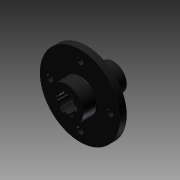
# Autodesk Inventor part: Denso-6
Saved by Autodesk Inventor 2011 (Build 150239000, 239)
## iProperties
Shininess: 64.0
Length Units: 11272
Angle Units: 11279
Time Units: 11290
Mass Units: 11286
Length Display Precision: 3
Angle Display Precision: 2
Category: Motors
Created: 2007-12-05
Material: ABS Plastic
Document SubType Name: Modeling
Density: 1 g/cm^3
Project: FIRST
Description: Coupler for Denso 6 Tooth Motor
Vendor: Pelham Plastics
Part Number: Denso-6
Density: 0.0
Volumn: 0.0
Area: 0.0
PropertySet Name: Model Information
Control State: 0
Master: False
Checked Out: False
Title: Coupler, Denso 6 tooth
Author: Autodesk, Inc.
Autodesk Inventor part; units mm, degrees
ref_plane "YZ Plane" through (0, 0, 0) normal (1, 0, 0) x (0, 1, 0)
ref_plane "XZ Plane" through (0, 0, 0) normal (0, 1, 0) x (-1, 0, 0)
ref_plane "XY Plane" through (0, 0, 0) normal (0, 0, 1) x (1, 0, 0)
sketch "Sketch1" plane through (0, 0, 0) normal (0, 0, 1) x (1, 0, 0)
  circle A0 centre (0, 0) radius 38.1
  dimension "d2" = 76.2
  constraints: 1 centre point
  measures "d2" diameter of A0
extrude "Extrusion1" add sketch "Sketch1" along normal mid plane 6.35
sketch "Sketch2" plane through (0, 0, 3.175) normal (0, 0, 1) x (1, 0, 0)
  circle A0 centre (0, 0) radius 38.1 projected
  point P0 (0, 28.575)
  dimension "d3" = 0
  dimension "d4" = 28.575
  measures "d3" horizontal distance of A0.centre point (0, 28.575)
  measures "d4" distance of A0.centre point (0, 28.575)
hole "Mounting Hole" at (0, 28.575, 3.175) direction (0, 0, -1) diameter 6.35 end through all
pattern_circular "Circular Pattern1" count 4 over 360 about axis through (0, 0, 0) along (0, 0, 1) of "Mounting Hole"
sketch "Sketch3" plane through (0, 0, 3.175) normal (0, 0, 1) x (1, 0, 0)
  circle A0 centre (0, 0) radius 38.1 projected
  circle A1 centre (0, 0) radius 15.875
  dimension "d15" = 31.75
  constraints: 1 centre point, 1 coincident
  measures "d15" diameter of A1
extrude "Extrusion2" add sketch "Sketch3" along normal blind 12.7 contours A1
sketch "Sketch8" plane through (0, 0, 15.875) normal (0, 0, 1) x (1, 0, 0)
  circle A0 centre (0, 0) radius 15.875 projected
  constraints: 1 coincident
hole "Hole3" at (0, 0, 15.875) direction (0, 0, -1) diameter 16.2 depth 14.986
sketch "Sketch4" plane through (0, 0, 15.875) normal (0, 0, 1) x (1, 0, 0)
  arc A0 (-3.0359, 9.528) -> (-6.5275, 7.5757) centre (0, 0) ccw
  circle A1 centre (0, 0) radius 15.875 projected
  line L0 (0, 0) -> (-5, 8.6603) construction
  line L1 (0, 0) -> (-10.16, 0) construction
  line L2 (-2.058, 7.8342) -> (-3.0359, 9.528)
  line L3 (-5.5564, 5.8937) -> (-6.5275, 7.5757)
  arc A2 (-2.058, 7.8342) -> (-5.5564, 5.8937) centre (0, 0) ccw
  circle A3 centre (0, 0) radius 8.1 projected
  dimension "d46" = 60
  dimension "d47" = 4
  dimension "d48" = 20
  constraints: 9 end point, 7 point on circle, 2 centre point, 2 parallel, 1 coincident, 1 concentric, 1 horizontal
  measures "d46" angle of L1 L0
  measures "d47" distance between parallel lines of L2 L3
  measures "d48" diameter of A0
extrude "Extrusion3" cut sketch "Sketch4" against normal up to surface (14.986 mm away) contours L2 A2 L3 A0
pattern_circular "Circular Pattern2" count 6 over 360 about axis through (0, 0, 0) along (0, 0, 1) of "Extrusion3"
sketch "Sketch5" plane through (0, 0, -3.175) normal (0, 0, -1) x (-1, 0, 0)
  circle A0 centre (0, 0) radius 38.1 projected
  circle A1 centre (0, 0) radius 14.9225
  dimension "d27" = 29.845
  constraints: 1 centre point, 1 coincident
  measures "d27" diameter of A1
extrude "Extrusion4" add sketch "Sketch5" along normal blind 25.4 draft -5 contours A1
sketch "Sketch6" plane through (0, 0, -28.575) normal (0, 0, -1) x (-1, 0, 0)
  circle A0 centre (0, 0) radius 12.7003 projected
  arc A1 (2.3812, -7.6374) -> (-2.3813, -7.6374) centre (0, 0) ccw
  line L0 (-2.3813, -7.6374) -> (-2.3812, -10.3188)
  line L1 (-2.3812, -10.3188) -> (2.3813, -10.3188)
  line L2 (2.3813, -10.3188) -> (2.3812, -7.6374)
  dimension "d31" = 16
  dimension "d32" = 4.7625
  dimension "d33" = 10.3187
  constraints: 6 end point, 2 parallel, 2 point on circle, 1 centre point, 1 coincident, 1 perpendicular, 1 vertical
  measures "d31" diameter of A1
  measures "d32" distance of L0.end L1.end
  measures "d33" distance from line of L1 A0.centre
extrude "Extrusion5" cut sketch "Sketch6" against normal blind 28.575 contours L2 L1 L0 A1
sketch "Sketch7" plane through (0, 0, 0) normal (0, 0, -1) x (-1, 0, 0)
  arc A0 (2.3812, -7.6374) -> (-2.3813, -7.6374) centre (0, 0) ccw projected
  point P0 (0, 0)
  constraints: 1 coincident
hole "Hole2" at (0, 0, 0) direction (0, 0, 1) diameter 9.525 end through all
fillet "Fillet1" radius 0.508 2 edges at (14.9225, 0, -3.175) (-15.875, 0, 3.175)
body "Solid1"
